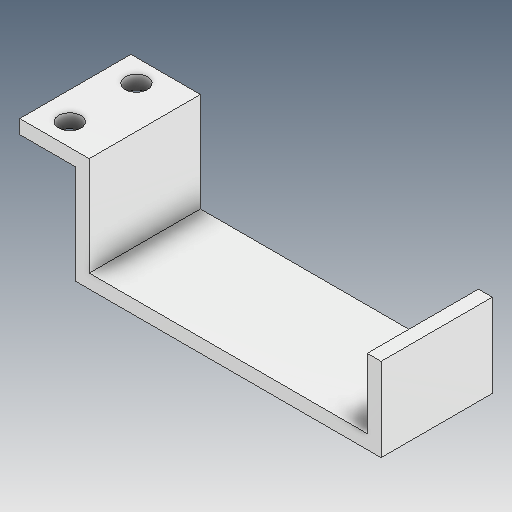
# Autodesk Inventor part: Carcasa para Placa Reed Switch 40x20
Saved by Autodesk Inventor 2020 (Build 240168000, 168)
## iProperties
Created: 2020-10-02
Part Number: Carcasa para Placa Reed Switch 40x20
Material: ABS Plastic
Document SubType Name: Modeling
Designer: Hernan
Density: 1.06 g/cm^3
Appearance: Smooth - White
Author: Hernan
Autodesk Inventor part; units mm, degrees
ref_plane "YZ Plane" through (0, 0, 0) normal (1, 0, 0) x (0, 1, 0)
ref_plane "XZ Plane" through (0, 0, 0) normal (0, 1, 0) x (-1, 0, 0)
ref_plane "XY Plane" through (0, 0, 0) normal (0, 0, 1) x (1, 0, 0)
sketch "Sketch1" plane through (0, 0, 0) normal (0, 0, 1) x (1, 0, 0)
  line L0 (-100.782, -11.9876) -> (-90.782, -11.9876)
  line L1 (-100.782, -9.4876) -> (-88.282, -9.4876)
  line L2 (-90.782, -11.9876) -> (-90.782, -20.4134)
  line L3 (-88.282, -9.4876) -> (-88.282, -20.4134)
  line L4 (-90.782, -20.4134) -> (-90.782, -29.8154)
  line L5 (-90.782, -29.8154) -> (-35.782, -29.8154)
  line L6 (-35.782, -29.8154) -> (-35.782, -14.8154)
  line L7 (-38.282, -14.8154) -> (-38.282, -27.3154)
  line L8 (-38.282, -27.3154) -> (-88.282, -27.3154)
  line L9 (-88.282, -27.3154) -> (-88.282, -20.4134)
  line L10 (-100.782, -11.9876) -> (-100.782, -9.4876)
  line L11 (-35.782, -14.8154) -> (-38.282, -14.8154)
  dimension "d6" = 10
  dimension "d7" = 2.5
  dimension "d8" = 2.5
  dimension "d9" = 2.5
  dimension "d20" = 15
  dimension "d21" = 65
  dimension "d29" = 2.5
  constraints: 24 end point, 5 perpendicular, 3 vertical, 2 horizontal
  measures "d6" distance of L0.start L0.end
  measures "d7" distance between parallel lines of L3 L2
  measures "d8" distance between parallel lines of L5 L8
  measures "d9" distance between parallel lines of L6 L7
  measures "d20" distance between parallel lines of L5 L11
  measures "d21" distance between parallel lines of L6 L10
  measures "d29" distance between parallel lines of L1 L0
extrude "Extrusion1" add sketch "Sketch1" along normal blind 20
sketch "Sketch2" plane through (-100.782, -11.9876, 0) normal (0, -1, 0) x (1, 0, 0)
  line L0 (0, 0) -> (0, 20) projected
  line L1 (10, 0) -> (10, 20) projected
  line L2 (0, 20) -> (10, 20) projected
  line L3 (0, 0) -> (10, 0) projected
  circle A0 centre (5, 4) radius 2
  circle A1 centre (5, 16) radius 2
  line L4 (65, 0) -> (65, 20) projected
  point P0 (100.782, 0)
  dimension "d17" = 4
  dimension "d22" = 4
  dimension "d24" = 12
  dimension "d25" = 4
  dimension "d27" = 60
  dimension "d28" = 60
  constraints: 2 centre point
  measures "d17" diameter of A1
  measures "d22" diameter of A0
  measures "d24" distance of A1.centre A0.centre
  measures "d25" distance from line of L2 A1.centre
  measures "d27" distance from line of L4 A0.centre
  measures "d28" distance from line of L4 A1.centre
extrude "Extrusion2" cut sketch "Sketch2" against normal blind 4 contours A0 | A1
equation "\"d17\" = d22"
body "Solid1"
